robot-before-lift-2026-10-04 (Autodesk Fusion 360 design; units mm, degrees)
Autodesk Fusion 360 part; units mm, degrees
sketch "Layout_Side" plane through (0, 0, 0) normal (0, 1, 0) x (1, 0, 0) in component "00_Layout"
  line L0 (0, 0) -> (0, -1676.4) construction
  line L1 (300, -275) -> (-300, -275) construction
  line L2 (-300, -275) -> (-300, -75) construction
  line L3 (-300, -75) -> (300, -75) construction
  line L4 (300, -75) -> (300, -275) construction
  line L5 (300, -275) -> (-300, -75) construction
  line L6 (-300, -275) -> (300, -75) construction
  line L7 (0, -1676.4) -> (600, -1676.4) construction
  line L8 (0, -175) -> (0, -75) construction
  dimension "d1" = 200
  dimension "d2" = 600
  dimension "d4" = 600
  dimension "d5" = 75
  dimension "d6" = 1676.4
  constraint vertical L0
  constraint horizontal L1
  constraint perpendicular L1 L2
  constraint parallel L1 L3
  constraint parallel L2 L4
  constraint perpendicular L0 L7
  constraint midpoint L3 L8.end
  constraint coincident L0.start origin
  constraint midpoint L8.start L5
  measures "d1" distance of L1.end L2.end
  measures "d2" distance of L1.start L1.end
  measures "d4" distance of L0.end L7.end
  measures "d5" distance of L0.start L8.end
  measures "d6" distance of L0.end L0.start
sketch "Base_Profile" plane through (0, 0, 0) normal (0, 1, 0) x (1, 0, 0) in component "01_Base_Envelope"
  line L0 (300, -275) -> (-300, -275)
  line L1 (-300, -275) -> (-300, -75)
  line L2 (-300, -75) -> (300, -75)
  line L3 (300, -75) -> (300, -275)
extrude "Chassis_Width_450mm" add sketch "Base_Profile" along normal mid plane 450 in component "01_Base_Envelope"
component "00_Layout" placed x (1, 0, 0) y (0, 1, 0) z (0, 0, 1) at (0, 0, 0)
component "01_Base_Envelope" placed x (1, 0, 0) y (0, 1, 0) z (0, 0, 1) at (0, 0, 0)
named bodies: "Chassis_Envelope"
